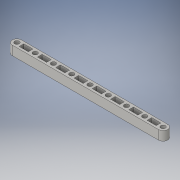
# Autodesk Inventor part: 8M Module
Saved by Autodesk Inventor 2016 SP1 (Build 200210100, 210)
## iProperties
Created: 2016-02-02
Part Number: 8M Module
Material: Wood (Cherry)
Document SubType Name: Modeling
Designer: jleonard
Density: 0.63 g/cm^3
Appearance: Cherry - Natural Low Gloss
Author: jleonard
Autodesk Inventor part; units mm, degrees
ref_plane "YZ Plane" through (0, 0, 0) normal (1, 0, 0) x (0, 1, 0)
ref_plane "XZ Plane" through (0, 0, 0) normal (0, 1, 0) x (-1, 0, 0)
ref_plane "XY Plane" through (0, 0, 0) normal (0, 0, 1) x (1, 0, 0)
sketch "Sketch1" plane through (0, 0, 0) normal (0, 1, 0) x (-1, 0, 0)
  line L0 (101.6, 6.35) -> (-101.6, 6.35)
  line L1 (-101.6, -6.35) -> (101.6, -6.35)
  arc A0 (101.6, -6.35) -> (101.6, 6.35) centre (101.6, 0) ccw
  arc A1 (-101.6, 6.35) -> (-101.6, -6.35) centre (-101.6, 0) ccw
  line L2 (151.13, 0) -> (-151.13, 0) projected
  line L3 (0, -8.89) -> (0, 8.89) projected
  point P0 (0, 0)
  dimension "d2" = 203.2
  dimension "d3" = 6.35
  dimension "d4" = 6.35
  dimension "d5" = 101.6
  dimension "d6" = 0
  dimension "d7" = 12.7
  dimension "d9" = 6.35
  dimension "d37" = 203.2
  constraints: 4 end point, 4 point on circle, 2 centre point, 1 horizontal, 1 parallel
  measures "d2" distance of A1.centre A0.centre
  measures "d3" radius of A1
  measures "d4" radius of A0
  measures "d5" distance from line of A1.centre L3
  measures "d6" distance from line of L2 A1.centre
  measures "d7" distance between parallel lines of L1 L0
  measures "d9" distance from line of L1 A0.centre
  measures "d37" distance of L0.start L0.end
extrude "Extrusion1" add sketch "Sketch1" along normal blind 12.7
sketch "Sketch4" plane through (0, 12.7, 0) normal (0, 1, 0) x (1, 0, 0)
  circle A0 centre (-101.6, 0) radius 3.175
  line L0 (-151.13, 0) -> (151.13, 0) projected
  line L1 (0, 8.89) -> (0, -8.89) projected
  circle A1 centre (-76.2, 0) radius 3.175
  circle A2 centre (-50.8, 0) radius 3.175
  circle A3 centre (-25.4, 0) radius 3.175
  circle A4 centre (0, 0) radius 3.175
  circle A5 centre (25.4, 0) radius 3.175
  circle A6 centre (50.8, 0) radius 3.175
  circle A7 centre (76.2, 0) radius 3.175
  circle A8 centre (101.6, 0) radius 3.175
  dimension "d45" = 6.35
  dimension "d46" = 101.6
  dimension "d47" = 0
  dimension "d50" = 25.4
  constraints: 9 centre point, 1 horizontal, 16 other
  measures "d45" diameter of A0
  measures "d46" distance from line of L1 A0.centre
  measures "d47" distance from line of L0 A0.centre
  measures "d50" distance of A0.centre A1.centre
extrude "Extrusion4" cut sketch "Sketch4" against normal through all
sketch "Sketch5" plane through (0, 12.7, 0) normal (0, 1, 0) x (1, 0, 0)
  line L0 (-95.25, -3.175) -> (-82.55, -3.175)
  line L1 (-82.55, -3.175) -> (-82.55, 3.175)
  line L2 (-82.55, 3.175) -> (-95.25, 3.175)
  line L3 (-95.25, 3.175) -> (-95.25, -3.175)
  line L4 (-151.13, 0) -> (151.13, 0) projected
  line L5 (0, 13.6448) -> (0, -37.419) projected
  line L6 (-57.15, 3.175) -> (-69.85, 3.175)
  line L7 (-69.85, 3.175) -> (-69.85, -3.175)
  line L8 (-69.85, -3.175) -> (-57.15, -3.175)
  line L9 (-57.15, -3.175) -> (-57.15, 3.175)
  line L10 (-31.75, 3.175) -> (-44.45, 3.175)
  line L11 (-44.45, 3.175) -> (-44.45, -3.175)
  line L12 (-44.45, -3.175) -> (-31.75, -3.175)
  line L13 (-31.75, -3.175) -> (-31.75, 3.175)
  line L14 (-6.35, 3.175) -> (-19.05, 3.175)
  line L15 (-19.05, 3.175) -> (-19.05, -3.175)
  line L16 (-19.05, -3.175) -> (-6.35, -3.175)
  line L17 (-6.35, -3.175) -> (-6.35, 3.175)
  line L18 (19.05, 3.175) -> (6.35, 3.175)
  line L19 (6.35, 3.175) -> (6.35, -3.175)
  line L20 (6.35, -3.175) -> (19.05, -3.175)
  line L21 (19.05, -3.175) -> (19.05, 3.175)
  line L22 (44.45, 3.175) -> (31.75, 3.175)
  line L23 (31.75, 3.175) -> (31.75, -3.175)
  line L24 (31.75, -3.175) -> (44.45, -3.175)
  line L25 (44.45, -3.175) -> (44.45, 3.175)
  line L26 (69.85, 3.175) -> (57.15, 3.175)
  line L27 (57.15, 3.175) -> (57.15, -3.175)
  line L28 (57.15, -3.175) -> (69.85, -3.175)
  line L29 (69.85, -3.175) -> (69.85, 3.175)
  line L30 (95.25, 3.175) -> (82.55, 3.175)
  line L31 (82.55, 3.175) -> (82.55, -3.175)
  line L32 (82.55, -3.175) -> (95.25, -3.175)
  line L33 (95.25, -3.175) -> (95.25, 3.175)
  point P0 (0, 0)
  dimension "d57" = 12.7
  dimension "d58" = 6.35
  dimension "d59" = 82.55
  dimension "d60" = 3.175
  dimension "d63" = 25.4
  constraints: 64 end point, 2 horizontal, 2 parallel, 1 perpendicular, 56 other
  measures "d57" distance of L0.start L0.end
  measures "d58" distance of L0.end L1.end
  measures "d59" distance between parallel lines of L5 L1
  measures "d60" distance between parallel lines of L0 L4
  measures "d63" distance of L1.end L6.start
extrude "Extrusion5" cut sketch "Sketch5" against normal through all
body "Solid1"
